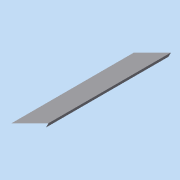
# Autodesk Inventor part: bottomplate
Saved by Autodesk Inventor 2016 (Build 200138000, 138)
## iProperties
Created: 2017-03-05
Part Number: bottomplate
Material: Generic
Document SubType Name: Modeling
Designer: Errrm
Density: 1 g/cm^3
Appearance: Default
Author: Errrm
Autodesk Inventor part; units mm, degrees
ref_plane "YZ Plane" through (0, 0, 0) normal (1, 0, 0) x (0, 1, 0)
ref_plane "XZ Plane" through (0, 0, 0) normal (0, 1, 0) x (-1, 0, 0)
ref_plane "XY Plane" through (0, 0, 0) normal (0, 0, 1) x (1, 0, 0)
sketch "Sketch1" plane through (0, 0, 0) normal (0, 0, 1) x (1, 0, 0)
  line L0 (0, 6) -> (50, 6) construction
  line L1 (50, -296) -> (0, -296) construction
  line L2 (0, 6) -> (38, 6)
  line L3 (38, 6) -> (38, -296)
  line L4 (38, -296) -> (0, -296)
  line L5 (0, -296) -> (0, 6)
  point P0 (19, -296)
  dimension "d2" = 38
  constraints: 8 end point, 2 parallel, 1 horizontal, 1 midpoint, 1 perpendicular, 1 point on line
  measures "d2" distance of L3.end L4.end
extrude "Extrusion1" add sketch "Sketch1" along normal blind 5
sketch "Sketch3" plane through (0, 0, 5) normal (0, 0, 1) x (1, 0, 0)
  circle A0 centre (12.5, -82.4963) radius 1 projected
  circle A1 centre (25.5, -82.4963) radius 1 projected
  circle A2 centre (12.5, -70.4963) radius 1 projected
  circle A3 centre (25.5, -70.4963) radius 1 projected
  circle A4 centre (25.5, -219.4963) radius 1 projected
  circle A5 centre (12.5, -219.4963) radius 1 projected
  circle A6 centre (12.5, -207.4963) radius 1 projected
  circle A7 centre (25.5, -207.4963) radius 1 projected
  point P0 (0, 0)
extrude "Extrusion2" cut sketch "Sketch3" against normal through all
body "Solid1"
